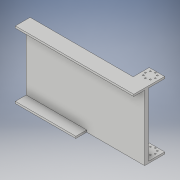
# Autodesk Inventor part: Guide
Saved by Autodesk Inventor 2019 (Build 230136000, 136)
## iProperties
Created: 2020-10-13
Part Number: Guide
Material: Generic
Document SubType Name: Modeling
Designer: Delta
Density: 1 g/cm^3
Appearance: Default
Author: Delta
Autodesk Inventor part; units mm, degrees
ref_plane "YZ Plane" through (0, 0, 0) normal (1, 0, 0) x (0, 1, 0)
ref_plane "XZ Plane" through (0, 0, 0) normal (0, 1, 0) x (-1, 0, 0)
sketch "Sketch1" plane through (0, 0, 0) normal (0, 0, 1) x (1, 0, 0)
  line L0 (0, 0) -> (233.68, 0)
  line L1 (233.68, 0) -> (233.68, 132.6642)
  line L2 (233.68, 132.6642) -> (0, 132.6642)
  line L3 (0, 132.6642) -> (0, 0)
  dimension "d0" = 132.6642
  dimension "d1" = 233.68
  constraints: 8 end point, 2 parallel, 1 horizontal, 1 perpendicular
  measures "d0" distance of L0.end L1.end
  measures "d1" distance of L1.end L2.end
extrude "Extrusion1" add sketch "Sketch1" along normal blind 29.21
sketch "Sketch2" plane through (0, 0, 29.21) normal (0, 0, 1) x (1, 0, 0)
  line L0 (-0.3825, 3.8354) -> (233.706, 3.8354)
  line L1 (233.706, 3.8354) -> (233.706, 128.8288)
  line L2 (233.706, 128.8288) -> (-0.3825, 128.8288)
  line L3 (-0.3825, 128.8288) -> (-0.3825, 3.8354)
  line L4 (233.68, 132.6642) -> (0, 132.6642) projected
  line L5 (0, 0) -> (233.68, 0) projected
  dimension "d4" = 3.8354
  dimension "d5" = 3.8354
  constraints: 8 end point, 2 parallel, 1 horizontal, 1 perpendicular
  measures "d4" distance between parallel lines of L4 L2
  measures "d5" distance between parallel lines of L5 L0
extrude "Extrusion2" cut sketch "Sketch2" against normal blind 21.4884
sketch "Sketch3" plane through (0, 0, 29.21) normal (0, 0, 1) x (1, 0, 0)
  line L0 (233.68, 0) -> (119.38, 0)
  line L1 (119.38, 0) -> (119.38, 3.8354)
  line L2 (119.38, 3.8354) -> (233.68, 3.8354)
  line L3 (233.68, 3.8354) -> (233.68, 0)
  point P0 (0, 0)
  dimension "d8" = 114.3
  dimension "d9" = 3.8354
  constraints: 8 end point, 2 parallel, 1 horizontal, 1 perpendicular
  measures "d8" distance of L1.end L2.end
  measures "d9" distance of L0.end L1.end
extrude "Extrusion3" cut sketch "Sketch3" against normal blind 21.4884
sketch "Sketch4" plane through (0, 0, 0) normal (0, 0, -1) x (-1, 0, 0)
  line L0 (-233.68, 0) -> (-233.68, 132.6642) projected
  line L1 (-233.68, 132.6642) -> (-203.2, 132.6642)
  line L2 (-203.2, 132.6642) -> (-203.2, 128.8288)
  line L3 (-203.2, 128.8288) -> (-233.68, 128.8288)
  line L4 (-233.68, 128.8288) -> (-233.68, 132.6642)
  line L5 (-233.68, 0) -> (-203.2, 0)
  line L6 (-203.2, 0) -> (-203.2, 3.8354)
  line L7 (-203.2, 3.8354) -> (-233.68, 3.8354)
  line L8 (-233.68, 3.8354) -> (-233.68, 0)
  point P0 (0, 0)
  dimension "d12" = 3.8354
  dimension "d13" = 30.48
  dimension "d14" = 3.8354
  dimension "d15" = 30.48
  constraints: 16 end point, 4 parallel, 2 horizontal, 2 perpendicular
  measures "d12" distance of L1.end L2.end
  measures "d13" distance of L2.end L3.end
  measures "d14" distance of L5.end L6.end
  measures "d15" distance of L6.end L7.end
extrude "Extrusion4" add sketch "Sketch4" along normal blind 31.75
sketch "Sketch7" plane through (0, 132.6642, 29.21) normal (0, 1, 0) x (1, 0, 0)
  circle A0 centre (217.8629, 48.5394) radius 2.54
  circle A1 centre (217.8134, 38.7605) radius 1.3589
  circle A2 centre (224.7426, 41.5897) radius 1.3589
  circle A3 centre (227.6418, 48.4899) radius 1.3589
  circle A4 centre (224.8126, 55.4191) radius 1.3589
  circle A5 centre (217.9124, 58.3182) radius 1.3589
  circle A6 centre (210.9832, 55.4891) radius 1.3589
  circle A7 centre (208.084, 48.5889) radius 1.3589
  circle A8 centre (210.9132, 41.6597) radius 1.3589
  point P0 (0, 29.21)
  dimension "d39" = 5.08
  dimension "d40" = 2.7178
  dimension "d41" = 9.779
  dimension "d44" = 360
  constraints: 9 centre point, 17 other
  measures "d39" diameter of A0
  measures "d40" diameter of A1
  measures "d41" distance of A1.centre A0.centre
extrude "Extrusion7" cut sketch "Sketch7" against normal blind 12.7 contours A1 | A2 | A3 | A4 | A5 | A6 | A7 | A8
ref_plane "Work Plane1" through (0, 66.3321, 0) normal (0, -1, 0) x (1, 0, 0)
mirror "Mirror2" about plane through (0, 66.3321, 0) normal (0, -1, 0) of "Extrusion7"
sketch "Sketch9" plane through (0, 0, 0) normal (0, -1, 0) x (1, 0, 0)
  circle A0 centre (157.48, 2.6482) radius 1.3589
  circle A1 centre (176.9362, 2.7347) radius 1.3589
  line L0 (119.38, 7.7216) -> (119.38, 29.21) projected
  point P0 (0, 0)
  dimension "d57" = 2.7178
  dimension "d58" = 19.4564
  dimension "d59" = 2.7178
  dimension "d60" = 38.1
  constraints: 2 centre point
  measures "d57" diameter of A0
  measures "d58" distance of A1.centre A0.centre
  measures "d59" diameter of A1
  measures "d60" distance from line of L0 A0.centre
extrude "Extrusion9" cut sketch "Sketch9" against normal blind 12.7
body "Solid1"
